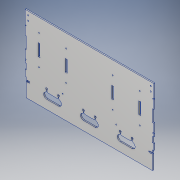
# Autodesk Inventor part: Hopper Side
Saved by Autodesk Inventor 2018 (Build 220112000, 112)
## iProperties
Created: 2013-10-08
Part Number: Hopper Side
Material: Aluminum 6061
Document SubType Name: Modeling
Designer: Gabriel Smolnycki
Mass: 1125.92 g
Surface Area: 2189.72 cm^2
Volume: 417.008 cm^3
Density: 2.7 g/cm^3
Appearance: Aluminum - Flat
Sending System: SolidWorks 2017
Last Author: Gabriel Smolnycki
Last Saved: 2017-09-14
Author: Gabriel Smolnycki
Autodesk Inventor part; units mm, degrees
ref_plane "YZ Plane" through (0, 0, 0) normal (1, 0, 0) x (0, 1, 0)
ref_plane "XZ Plane" through (0, 0, 0) normal (0, 1, 0) x (-1, 0, 0)
ref_plane "Work Plane1" through (0, 0, -4) normal (0, 0, 1) x (1, 0, 0)
sketch "Sketch1" plane through (0, 0, -4) normal (0, 0, 1) x (1, 0, 0)
  line L0 (165.85, 12.5) -> (172.15, 12.5)
  line L1 (209, -79.25) -> (212, -79.25)
  line L2 (-212, -127.5) -> (212, -127.5)
  line L3 (216, 84.25) -> (214, 84.25)
  arc A0 (21.9244, -70.119) -> (17.7103, -69.8065) centre (20, -67.5) ccw
  arc A1 (-108.9601, -77.5) -> (-105.7897, -69.8065) centre (-108.9601, -73) ccw
  line L4 (-209, -74.75) -> (-209, -75.75)
  line L5 (216, -27.5) -> (216, -19.25)
  arc A2 (145.4244, -70.119) -> (141.2103, -69.8065) centre (143.5, -67.5) ccw
  arc A3 (14.5399, -77.5) -> (17.7103, -69.8065) centre (14.5399, -73) ccw
  line L6 (-108.9601, -77.5) -> (-138.0399, -77.5)
  line L7 (74.85, 52.5) -> (74.85, 12.5)
  line L8 (-209, -75.75) -> (-212, -75.75)
  arc A4 (-214, 80.75) -> (-214, 84.25) centre (-214, 82.5) ccw
  line L9 (216, -27.5) -> (212, -27.5)
  line L10 (-216, -19.25) -> (-216, -27.5)
  arc A5 (-141.2103, -69.8065) -> (-138.0399, -77.5) centre (-138.0399, -73) ccw
  line L11 (74.85, 12.5) -> (81.15, 12.5)
  line L12 (-212, -75.75) -> (-212, -67)
  line L13 (-214, 84.25) -> (-216, 84.25)
  line L14 (212, -27.5) -> (212, -46.5)
  line L15 (-216, -19.25) -> (-214, -19.25)
  arc A6 (138.0399, -77.5) -> (141.2103, -69.8065) centre (138.0399, -73) ccw
  arc A7 (-141.2103, -69.8065) -> (-145.4244, -70.119) centre (-143.5, -67.5) ccw
  line L16 (81.15, 12.5) -> (81.15, 52.5)
  line L17 (-216, -67) -> (-212, -67)
  line L18 (-216, 127.5) -> (-216, 84.25)
  line L19 (216, -46.5) -> (212, -46.5)
  line L20 (81.15, 52.5) -> (74.85, 52.5)
  line L21 (138.0399, -77.5) -> (108.9601, -77.5)
  arc A8 (-146.6648, -78.014) -> (-145.4244, -70.119) centre (-148.089, -73.7453) ccw
  line L22 (-216, -46.5) -> (-216, -67)
  line L23 (216, 127.5) -> (-216, 127.5)
  line L24 (216, -67) -> (216, -46.5)
  arc A9 (105.7897, -69.8065) -> (108.9601, -77.5) centre (108.9601, -73) ccw
  line L25 (212, -79.25) -> (212, -127.5)
  line L26 (-212, -46.5) -> (-216, -46.5)
  line L27 (216, 84.25) -> (216, 127.5)
  line L28 (212, -67) -> (216, -67)
  arc A10 (105.7897, -69.8065) -> (101.5756, -70.119) centre (103.5, -67.5) ccw
  line L29 (-172.15, 12.5) -> (-165.85, 12.5)
  line L30 (-212, -46.5) -> (-212, -27.5)
  line L31 (212, -67) -> (212, -75.75)
  arc A11 (100.3352, -78.014) -> (101.5756, -70.119) centre (98.911, -73.7453) ccw
  line L32 (-165.85, 12.5) -> (-165.85, 52.5)
  line L33 (-212, -127.5) -> (-212, -79.25)
  line L34 (-212, -27.5) -> (-216, -27.5)
  arc A12 (214, 84.25) -> (214, 80.75) centre (214, 82.5) ccw
  line L35 (212, -75.75) -> (209, -75.75)
  line L36 (14.5399, -77.5) -> (-14.5399, -77.5)
  arc A13 (100.3352, -78.014) -> (103.5, -97.5) centre (103.5, -87.5) ccw
  line L37 (-165.85, 52.5) -> (-172.15, 52.5)
  line L38 (-212, -79.25) -> (-209, -79.25)
  line L39 (214, 80.75) -> (216, 80.75)
  line L40 (209, -75.75) -> (209, -74.75)
  line L41 (216, -15.75) -> (214, -15.75)
  line L42 (103.5, -97.5) -> (143.5, -97.5)
  line L43 (-209, -79.25) -> (-209, -80.25)
  line L44 (216, 52.5) -> (216, 80.75)
  line L45 (209, -74.75) -> (205, -74.75)
  line L46 (-172.15, 52.5) -> (-172.15, 12.5)
  arc A14 (-17.7103, -69.8065) -> (-14.5399, -77.5) centre (-14.5399, -73) ccw
  arc A15 (143.5, -97.5) -> (146.6648, -78.014) centre (143.5, -87.5) ccw
  line L47 (-81.15, 12.5) -> (-74.85, 12.5)
  line L48 (-209, -80.25) -> (-205, -80.25)
  arc A16 (-214, -19.25) -> (-214, -15.75) centre (-214, -17.5) ccw
  line L49 (216, 52.5) -> (212, 52.5)
  line L50 (205, -74.75) -> (205, -75.75)
  line L51 (-216, 80.75) -> (-214, 80.75)
  arc A17 (-146.6648, -78.014) -> (-143.5, -97.5) centre (-143.5, -87.5) ccw
  arc A18 (-17.7103, -69.8065) -> (-21.9244, -70.119) centre (-20, -67.5) ccw
  arc A19 (145.4244, -70.119) -> (146.6648, -78.014) centre (148.089, -73.7453) ccw
  line L52 (-74.85, 12.5) -> (-74.85, 52.5)
  line L53 (-205, -80.25) -> (-205, -79.25)
  line L54 (-214, -15.75) -> (-216, -15.75)
  line L55 (212, 52.5) -> (212, 12.5)
  line L56 (205, -75.75) -> (200, -75.75)
  arc A20 (-23.1648, -78.014) -> (-21.9244, -70.119) centre (-24.589, -73.7453) ccw
  line L57 (-74.85, 52.5) -> (-81.15, 52.5)
  line L58 (-205, -79.25) -> (-200, -79.25)
  line L59 (-216, 12.5) -> (-216, -15.75)
  line L60 (212, 12.5) -> (216, 12.5)
  line L61 (200, -75.75) -> (200, -79.25)
  line L62 (-81.15, 52.5) -> (-81.15, 12.5)
  arc A21 (-23.1648, -78.014) -> (-20, -97.5) centre (-20, -87.5) ccw
  line L63 (-143.5, -97.5) -> (-103.5, -97.5)
  line L64 (-200, -79.25) -> (-200, -75.75)
  line L65 (-216, 12.5) -> (-212, 12.5)
  line L66 (216, -15.75) -> (216, 12.5)
  line L67 (200, -79.25) -> (205, -79.25)
  line L68 (-20, -97.5) -> (20, -97.5)
  arc A22 (-103.5, -97.5) -> (-100.3352, -78.014) centre (-103.5, -87.5) ccw
  line L69 (172.15, 12.5) -> (172.15, 52.5)
  line L70 (-200, -75.75) -> (-205, -75.75)
  line L71 (-212, 12.5) -> (-212, 52.5)
  line L72 (205, -79.25) -> (205, -80.25)
  arc A23 (20, -97.5) -> (23.1648, -78.014) centre (20, -87.5) ccw
  arc A24 (-101.5756, -70.119) -> (-100.3352, -78.014) centre (-98.911, -73.7453) ccw
  line L73 (172.15, 52.5) -> (165.85, 52.5)
  line L74 (-205, -75.75) -> (-205, -74.75)
  line L75 (-212, 52.5) -> (-216, 52.5)
  arc A25 (214, -15.75) -> (214, -19.25) centre (214, -17.5) ccw
  line L76 (205, -80.25) -> (209, -80.25)
  arc A26 (21.9244, -70.119) -> (23.1648, -78.014) centre (24.589, -73.7453) ccw
  arc A27 (-101.5756, -70.119) -> (-105.7897, -69.8065) centre (-103.5, -67.5) ccw
  line L77 (165.85, 52.5) -> (165.85, 12.5)
  line L78 (-205, -74.75) -> (-209, -74.75)
  line L79 (-216, 80.75) -> (-216, 52.5)
  line L80 (214, -19.25) -> (216, -19.25)
  line L81 (209, -80.25) -> (209, -79.25)
  constraints: 164 end point, 56 point on circle, 46 horizontal, 44 equal length, 36 vertical, 28 centre point, 25 collinear
extrude "Extrusion1" add sketch "Sketch1" along normal blind 4.064
hole "Hole14" at (-205.5, 115.5, 0) direction (0, 0, -1) diameter 4.5 depth 4
hole "Hole13" at (-205.5, 99.5, 0) direction (0, 0, -1) diameter 4.5 depth 4
hole "Hole12" at (205.5, 99.5, 0) direction (0, 0, -1) diameter 4.5 depth 4
hole "Hole11" at (205.5, 115.5, 0) direction (0, 0, -1) diameter 4.5 depth 4
hole "Hole10" at (90, -54.5, -4) direction (0, 0, 1) diameter 3.5 depth 4.064
hole "Hole9" at (-90, -54.5, -4) direction (0, 0, 1) diameter 3.5 depth 4.064
hole "Hole8" at (78, 82.5, -4) direction (0, 0, 1) diameter 3.5 depth 4.064
sketch "Sketch8" plane through (0, 0, -4) normal (0, 0, 1) x (1, 0, 0)
  point P0 (78, 82.5)
hole "Hole7" at (78, -17.5, -4) direction (0, 0, 1) diameter 3.5 depth 4.064
sketch "Sketch7" plane through (0, 0, -4) normal (0, 0, 1) x (1, 0, 0)
  point P0 (-90, -54.5)
hole "Hole6" at (169, -17.5, -4) direction (0, 0, 1) diameter 3.5 depth 4.064
sketch "Sketch6" plane through (0, 0, -4) normal (0, 0, 1) x (1, 0, 0)
  point P0 (90, -54.5)
hole "Hole5" at (169, 82.5, -4) direction (0, 0, 1) diameter 3.5 depth 4.064
sketch "Sketch5" plane through (0, 0, 0) normal (0, 0, 1) x (1, 0, 0)
  point P0 (205.5, 115.5)
hole "Hole4" at (-169, -17.5, -4) direction (0, 0, 1) diameter 3.5 depth 4.064
sketch "Sketch4" plane through (0, 0, 0) normal (0, 0, 1) x (1, 0, 0)
  point P0 (205.5, 99.5)
hole "Hole3" at (-78, -17.5, -4) direction (0, 0, 1) diameter 3.5 depth 4.064
sketch "Sketch3" plane through (0, 0, 0) normal (0, 0, 1) x (1, 0, 0)
  point P0 (-205.5, 99.5)
hole "Hole2" at (-78, 82.5, -4) direction (0, 0, 1) diameter 3.5 depth 4.064
sketch "Sketch2" plane through (0, 0, 0) normal (0, 0, 1) x (1, 0, 0)
  point P0 (-205.5, 115.5)
hole "Hole1" at (-169, 82.5, -4) direction (0, 0, 1) diameter 3.5 depth 4.064
sketch "Sketch9" plane through (0, 0, -4) normal (0, 0, 1) x (1, 0, 0)
  point P0 (78, -17.5)
sketch "Sketch10" plane through (0, 0, -4) normal (0, 0, 1) x (1, 0, 0)
  point P0 (169, -17.5)
sketch "Sketch11" plane through (0, 0, -4) normal (0, 0, 1) x (1, 0, 0)
  point P0 (169, 82.5)
sketch "Sketch12" plane through (0, 0, -4) normal (0, 0, 1) x (1, 0, 0)
  point P0 (-169, -17.5)
sketch "Sketch13" plane through (0, 0, -4) normal (0, 0, 1) x (1, 0, 0)
  point P0 (-78, -17.5)
sketch "Sketch14" plane through (0, 0, -4) normal (0, 0, 1) x (1, 0, 0)
  point P0 (-78, 82.5)
sketch "Sketch15" plane through (0, 0, -4) normal (0, 0, 1) x (1, 0, 0)
  point P0 (-169, 82.5)
body "Solid3"
